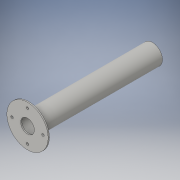
# Autodesk Inventor part: 40mm_flange
Saved by Autodesk Inventor 2016 (Build 200138000, 138)
## iProperties
Created: 2015-09-15
Part Number: 40mm_flange
Material: Generic
Document SubType Name: Modeling
Designer: KA ROSIE
Density: 1 g/cm^3
Appearance: Default
Author: KA ROSIE
Autodesk Inventor part; units mm, degrees
ref_plane "YZ Plane" through (0, 0, 0) normal (1, 0, 0) x (0, 1, 0)
ref_plane "XZ Plane" through (0, 0, 0) normal (0, 1, 0) x (-1, 0, 0)
ref_plane "XY Plane" through (0, 0, 0) normal (0, 0, 1) x (1, 0, 0)
ref_plane "Work Plane1" through (0, 0, 0) normal (0, 0, 1) x (1, 0, 0)
sketch "Sketch2" plane through (0, 0, 0) normal (0, 0, 1) x (1, 0, 0)
  circle A0 centre (0, 0) radius 16.75
  circle A1 centre (0, 0) radius 50
  point P0 (0, 0)
  dimension "d0" = 33.5
  dimension "d25" = 100
  constraints: 2 centre point, 2 coincident
  measures "d0" diameter of A0
  measures "d25" diameter of A1
extrude "Extrusion1" add sketch "Sketch2" along normal blind 3
sketch "Sketch3" plane through (0, 0, 0) normal (0, 0, -1) x (-1, 0, 0)
  circle A0 centre (0, 0) radius 24.25
  circle A1 centre (0, 0) radius 21.75
  point P0 (0, 0)
  dimension "d4" = 48.5
  dimension "d26" = 2.5
  constraints: 2 centre point, 1 coincident
  measures "d4" diameter of A0
  measures "d26" radial gap between concentric circles of A1 A0
extrude "Extrusion2" add sketch "Sketch3" along normal blind 300
sketch "Sketch4" plane through (0, 0, 0) normal (0, 0, -1) x (-1, 0, 0)
  circle A0 centre (0, 0) radius 16.75 projected
  circle A1 centre (0, 0) radius 37.5 construction
  circle A2 centre (37.5, 0) radius 3
  circle A3 centre (0, 0) radius 37.5 construction
  circle A4 centre (0, 37.5) radius 3
  circle A5 centre (0, 0) radius 37.5 construction
  circle A6 centre (-37.5, 0) radius 3
  circle A7 centre (0, 0) radius 37.5 construction
  circle A8 centre (0, -37.5) radius 3
  point P0 (0, 0)
  dimension "d9" = 75
  dimension "d10" = 6
  dimension "d13" = 360
  constraints: 4 centre point, 3 coincident, 2 horizontal alignment, 2 vertical alignment, 23 other
  measures "d10" diameter of A2
hole "Hole1" at (-37.5, 0, 0) at (0, -37.5, 0) at (37.5, 0, 0) at (0, 37.5, 0) direction (0, 0, 1) diameter 6 end through all
body "Solid1"
